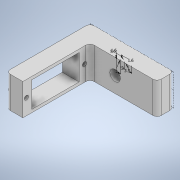
# Autodesk Inventor part: L-bracket
Saved by Autodesk Inventor 2022 (Build 260153000, 153)
## iProperties
Created: 2021-07-28
Part Number: L-bracket
Material: Generic
Document SubType Name: Modeling
Designer: WASHINGTON
Density: 1 g/cm^3
Appearance: Default
Author: WASHINGTON
Autodesk Inventor part; units mm, degrees
ref_plane "YZ Plane" through (0, 0, 0) normal (1, 0, 0) x (0, 1, 0)
ref_plane "XZ Plane" through (0, 0, 0) normal (0, 1, 0) x (-1, 0, 0)
ref_plane "XY Plane" through (0, 0, 0) normal (0, 0, 1) x (1, 0, 0)
sketch "Sketch1" plane through (0, 0, 0) normal (0, 1, 0) x (-1, 0, 0)
  line L0 (-2, 40) -> (-6, 40)
  line L1 (-8, 38) -> (-8, 10)
  line L2 (-8, 0) -> (-2, 0)
  line L3 (0, 2) -> (0, 38)
  line L4 (-8, 0) -> (-38, 0)
  line L5 (-40, 2) -> (-40, 6)
  line L6 (-38, 8) -> (-10, 8)
  arc A0 (-10, 8) -> (-8, 10) centre (-10, 10) ccw
  arc A1 (0, 38) -> (-2, 40) centre (-2, 38) ccw
  arc A2 (-38, 8) -> (-40, 6) centre (-38, 6) ccw
  arc A3 (-40, 2) -> (-38, 0) centre (-38, 2) ccw
  arc A4 (-2, 0) -> (0, 2) centre (-2, 2) ccw
  line L7 (-8, 38) -> (-8, 40)
  line L8 (-6, 40) -> (-8, 40)
  point P0 (0, 0)
  point P1 (0, 40)
  point P2 (0, 0)
  point P3 (-40, 8)
  point P4 (-40, 0)
  dimension "d0" = 2
  dimension "d1" = 40
  dimension "d2" = 40
  dimension "d3" = 8
  dimension "d4" = 8
  dimension "d5" = 8
  dimension "d6" = 32
  dimension "d7" = 0
  dimension "d8" = 2
  constraints: 18 end point, 10 point on circle, 10 point on line, 10 tangent, 5 centre point, 3 parallel, 3 perpendicular, 2 horizontal, 1 vertical
  measures "d0" radius of A0
  measures "d1" distance of point (0, 0) point (0, 40)
  measures "d2" distance of point (-40, 0) point (0, 0)
  measures "d3" distance of point (0, 40) L7.end
  measures "d4" distance of point (-40, 0) point (-40, 8)
  measures "d5" distance of L2.start point (0, 0)
  measures "d6" distance of L2.start point (-40, 0)
  measures "d7" distance from line of point (0, 0) L3
  measures "d8" radius of A1
extrude "Extrusion1" add sketch "Sketch1" along normal mid plane 15
sketch "Sketch2" plane through (10, 7.5, 8) normal (0, 0, 1) x (1, 0, 0)
  line L0 (-8, 0) -> (-10, 0) construction
  line L1 (30, -15) -> (30, 0) construction
  line L2 (-10, 0) -> (30, 0) construction
  line L3 (30, 0) -> (30, -15) construction
  line L4 (30, -15) -> (-10, -15) construction
  line L5 (-10, -15) -> (-10, 0) construction
  line L6 (30, 0) -> (28, 0) construction
  line L7 (-10, -15) -> (30, 0) construction
  line L8 (-10, -15) -> (-10, 0) construction
  line L9 (-10, 0) -> (30, -15) construction
  circle A0 centre (10, -7.5) radius 2.5
  point P0 (-10, -7.5)
  dimension "d11" = 5
  constraints: 12 end point, 2 parallel, 1 centre point, 1 horizontal, 1 midpoint, 1 perpendicular
  measures "d11" diameter of A0
hole "Hole1" at (20, 0, 8) direction (0, 0, -1) diameter 5 end through all
sketch "Sketch3" plane through (8, -7.5, 10) normal (1, 0, 0) x (0, 0, -1)
  line L0 (-28, 15) -> (-30, 15) construction
  line L1 (8, 0) -> (10, 0) construction
  line L2 (-30, 15) -> (10, 15) construction
  line L3 (10, 15) -> (10, 0) construction
  line L4 (10, 0) -> (-30, 0) construction
  line L5 (-30, 0) -> (-30, 15) construction
  line L6 (10, 0) -> (10, 15) construction
  line L7 (-30, 0) -> (10, 15) construction
  line L8 (-30, 0) -> (-30, 15) construction
  line L9 (10, 15) -> (-30, 15) construction
  line L10 (-30, 15) -> (10, 0) construction
  line L11 (-21.31, 1.39) -> (1.31, 1.39) construction
  line L12 (1.31, 1.39) -> (1.31, 13.61) construction
  line L13 (1.31, 13.61) -> (-21.31, 13.61) construction
  line L14 (-21.31, 13.61) -> (-21.31, 1.39) construction
  line L15 (-21.31, 1.39) -> (1.31, 13.61) construction
  line L16 (1.31, 1.39) -> (-21.31, 13.61) construction
  line L17 (-10, 7.5) -> (-34.1709, 7.5) construction
  line L18 (-3.19, 13.6) -> (-25.81, 13.6)
  line L19 (-25.81, 13.6) -> (-25.81, 1.4)
  line L20 (-25.81, 1.4) -> (-3.19, 1.4)
  line L21 (-3.19, 1.4) -> (-3.19, 13.6)
  line L22 (-3.19, 13.6) -> (-25.81, 1.4) construction
  line L23 (-25.81, 13.6) -> (-3.19, 1.4) construction
  point P0 (10, 7.5)
  point P1 (-14.5, 7.5)
  dimension "d19" = 22.62
  dimension "d20" = 12.22
  dimension "d21" = 22.62
  dimension "d22" = 12.2
  dimension "d23" = 4.5
  constraints: 40 end point, 6 parallel, 5 midpoint, 4 horizontal, 4 perpendicular, 1 point on line
  measures "d19" distance of L13.end L12.end
  measures "d20" distance of L12.end L11.end
  measures "d21" distance of L20.end L19.end
  measures "d22" distance of L19.end L18.end
  measures "d23" distance of L17.start point (-14.5, 7.5)
extrude "Extrusion2" cut sketch "Sketch3" against normal through all
sketch "Sketch4" plane through (8, -7.5, 10) normal (1, 0, 0) x (0, 0, -1)
  line L0 (-3.19, 13.6) -> (-25.81, 13.6) construction
  line L1 (-25.81, 1.4) -> (-3.19, 1.4) construction
  line L2 (-3.19, 1.4) -> (-3.19, 13.6) construction
  line L3 (-3.19, 13.6) -> (-25.81, 13.6) construction
  line L4 (-25.81, 13.6) -> (-25.81, 1.4) construction
  line L5 (-25.81, 1.4) -> (-3.19, 13.6) construction
  line L6 (-3.19, 1.4) -> (-25.81, 13.6) construction
  line L7 (-14.5, 7.5) -> (-36.2252, 7.5) construction
  line L8 (-36.2252, 7.5) -> (0.1, 7.5) construction
  circle A0 centre (-28.35, 7.5) radius 1
  circle A1 centre (-0.65, 7.5) radius 1
  point P0 (10, 7.5)
  dimension "d26" = 13.85
  dimension "d27" = 13.85
  dimension "d28" = 2
  dimension "d29" = 2
  dimension "d30" = 28.34
  dimension "d31" = 12.2
  dimension "d32" = 3.29
  dimension "d33" = 33.0352
  constraints: 16 end point, 3 point on line, 2 centre point, 2 horizontal, 2 midpoint, 2 parallel, 1 perpendicular
  measures "d26" distance of L7.start A0.centre
  measures "d27" distance of A1.centre L7.start
  measures "d28" diameter of A0
  measures "d29" diameter of A1
  measures "d30" angle of L5 L0
  measures "d31" distance between parallel lines of L1 L0
  measures "d32" distance from line of L8.end L2
  measures "d33" distance from line of L7.end L2
extrude "Extrusion3" cut sketch "Sketch4" along normal through all both and the other way through all
sketch "Sketch5" plane through (38, 7.5, 0) normal (0, 0, -1) x (-1, 0, 0)
  line L0 (-2, -15) -> (-2, 0) construction
  line L1 (36, -15) -> (38, -15) construction
  line L2 (-2, 0) -> (38, 0) construction
  line L3 (38, 0) -> (38, -15) construction
  line L4 (38, -15) -> (-2, -15) construction
  line L5 (-2, -15) -> (-2, 0) construction
  line L6 (-2, 0) -> (38, -15) construction
  line L7 (38, 0) -> (36, 0) construction
  line L8 (38, 0) -> (-2, -15) construction
  line L9 (-2, -7.5) -> (38, -7.5) construction
  circle A0 centre (21.5, -7.5) radius 0.8
  circle A1 centre (23.5, -7.5) radius 0.8
  circle A2 centre (25.5, -7.5) radius 0.8
  point P0 (18, -7.5)
  dimension "d36" = 1.6
  dimension "d37" = 1.6
  dimension "d38" = 1.6
  dimension "d39" = 2
  dimension "d40" = 2
  dimension "d41" = 3.5
  constraints: 14 end point, 3 centre point, 3 point on line, 2 horizontal, 2 midpoint, 2 parallel, 1 perpendicular
  measures "d36" diameter of A0
  measures "d37" diameter of A1
  measures "d38" diameter of A2
  measures "d39" distance of A1.centre A0.centre
  measures "d40" distance of A2.centre A1.centre
  measures "d41" distance of A0.centre point (18, -7.5)
body "Solid1"
